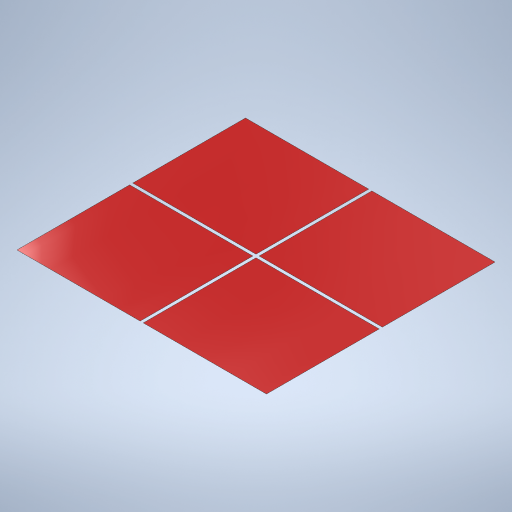
# Autodesk Inventor part: keepout - bottom
Saved by Autodesk Inventor 2023 (Build 270158000, 158)
## iProperties
Created: 2023-03-02
Part Number: keepout - bottom
Material: Generic
Document SubType Name: Modeling
Designer: Caleb
Density: 1 g/cm^3
Appearance: Default
Author: Caleb
Autodesk Inventor part; units mm, degrees
ref_plane "YZ Plane" through (0, 0, 0) normal (1, 0, 0) x (0, 1, 0)
ref_plane "XZ Plane" through (0, 0, 0) normal (0, 1, 0) x (-1, 0, 0)
ref_plane "XY Plane" through (0, 0, 0) normal (0, 0, 1) x (1, 0, 0)
sketch "Sketch1" plane through (0, 0, 0) normal (0, 1, 0) x (-1, 0, 0)
  line L0 (-23.8, -21.8) -> (23.8, -21.8)
  line L1 (23.8, -21.8) -> (23.8, 21.8)
  line L2 (23.8, 21.8) -> (-23.8, 21.8)
  line L3 (-23.8, 21.8) -> (-23.8, -21.8)
  line L4 (-23.8, -21.8) -> (23.8, 21.8) construction
  line L5 (23.8, -21.8) -> (-23.8, 21.8) construction
  point P0 (0, 0)
  dimension "d0" = 47.6
  dimension "d1" = 43.6
  constraints: 12 end point, 2 midpoint, 2 parallel, 1 horizontal, 1 perpendicular
  measures "d0" distance of L1.end L2.end
  measures "d1" distance of L0.end L1.end
extrude "Extrusion1" add sketch "Sketch1" along normal blind 0.01
sketch "Sketch2" plane through (0, 0.01, 0) normal (0, 1, 0) x (1, 0, 0)
  line L0 (-23.8, 21.8) -> (-23.8, -21.8) projected
  line L1 (23.8, 0.3) -> (-23.8, 0.3)
  line L2 (-23.8, 0.3) -> (-23.8, -0.3)
  line L3 (-23.8, -0.3) -> (23.8, -0.3)
  line L4 (23.8, -0.3) -> (23.8, 0.3)
  line L5 (23.8, 0.3) -> (-23.8, -0.3) construction
  line L6 (-23.8, 0.3) -> (23.8, -0.3) construction
  line L7 (-23.8, -21.8) -> (23.8, -21.8) projected
  line L8 (0.3, 21.8) -> (-0.3, 21.8)
  line L9 (-0.3, 21.8) -> (-0.3, -21.8)
  line L10 (-0.3, -21.8) -> (0.3, -21.8)
  line L11 (0.3, -21.8) -> (0.3, 21.8)
  line L12 (0.3, 21.8) -> (-0.3, -21.8) construction
  line L13 (-0.3, 21.8) -> (0.3, -21.8) construction
  point P0 (0, 0)
  point P1 (0.3, -0.3)
  point P2 (0.3, 0.3)
  point P3 (-0.3, 0.3)
  point P4 (-0.3, -0.3)
  dimension "d4" = 0.6
  dimension "d8" = 0.6
  constraints: 24 end point, 4 midpoint, 4 parallel, 2 horizontal, 2 perpendicular, 2 point on line
  measures "d4" distance between parallel lines of L3 L1
  measures "d8" distance between parallel lines of L11 L9
extrude "Extrusion2" cut sketch "Sketch2" against normal through all contours L1 L9 L3 L0 | L9 L8 L11 L1 | L1 L11 L3 L9 | L3 L11 L7 L9 | L1 L4 L3 L11
body "Solid1"
